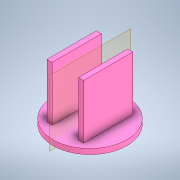
# Autodesk Inventor part: pvcBracketUpperPortionV02
Saved by Autodesk Inventor 2022.2 (Build 262287000, 287)
## iProperties
Created: 2021-10-20
Part Number: pvcBracketUpperPortionV02
Material: PC/ABS Plastic
Document SubType Name: Modeling
Designer: robst
Density: 0.357273 g/cm^3
Appearance: Pink
Author: robst
Autodesk Inventor part; units mm, degrees
ref_plane "XZ Plane" through (0, 0, 0) normal (0, 1, 0) x (-1, 0, 0)
ref_plane "XY Plane" through (0, 0, 0) normal (0, 0, 1) x (1, 0, 0)
sketch "Sketch51" plane through (0, 0, 0) normal (0, 1, 0) x (-1, 0, 0)
  circle A0 centre (0, 0) radius 57.15
  dimension "d242" = 114.3
  constraints: 1 centre point, 1 coincident
  measures "d242" diameter of A0
extrude "Extrusion26" add sketch "Sketch51" against normal blind 8
sketch "Sketch79" plane through (0, 0, 0) normal (0, 1, 0) x (1, 0, 0)
  line L0 (0, 0) -> (-57.15, 0) construction
  circle A0 centre (0, 0) radius 57.15 construction
  line L1 (-28.32, -38.1) -> (-20.32, -38.1)
  line L2 (-20.32, -38.1) -> (-20.32, 38.1)
  line L3 (-20.32, 38.1) -> (-28.32, 38.1)
  line L4 (-28.32, 38.1) -> (-28.32, -38.1)
  line L5 (-28.32, -38.1) -> (-20.32, 38.1) construction
  line L6 (-20.32, -38.1) -> (-28.32, 38.1) construction
  point P0 (-24.32, 0)
  dimension "d346" = 76.2
  dimension "d347" = 8
  dimension "d348" = 20.32
  constraints: 14 end point, 2 horizontal, 2 midpoint, 2 parallel, 1 horizontal alignment, 1 perpendicular, 1 point on line, 1 other
  measures "d346" distance of L3.end L1.start
  measures "d347" distance of L1.start L1.end
  measures "d348" distance from line of L2 L0.start
extrude "Extrusion31" add sketch "Sketch79" along normal blind 84.1375
mirror "Mirror4" about plane through (0, 0, 0) normal (1, 0, 0) of "Extrusion31"
equation "\"d243\" = wallThickness"
equation "\"wallThickness\" = 8"
equation "\"twoByFourWidth\" = 40.64"
equation "\"twoByFourDepth\" = 84.1375"
equation "\"azimuth\" = 55deg"
equation "\"elevationOfTwoByFour\" = 20deg"
equation "\"depthOfExtrusionForMatingToLowerHalf\" = 12.5"
equation "\"depthForWasherForMatingToCase\" = 14"
equation "\"pvcPipeInsideDiameter\" = 50.8"
equation "\"pvcPipeOutsideDiameter\" = 2.375"
equation "\"pvcPipeInsertDepth\" = 25"
equation "\"outsideDiameterOfBottom\" = 88.9"
equation "\"angleForGarage2x4\" = 20deg"
body "Solid4"
